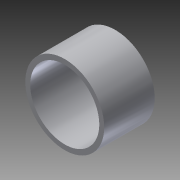
# Autodesk Inventor part: Spacer (0.4375 ID whatever OD) aluminum
Saved by Autodesk Inventor 2014 (Build 180170000, 170)
## iProperties
Created: 2014-01-20
Part Number: Spacer (0.4375 ID whatever OD) aluminum
Material: Aluminum 6061
Document SubType Name: Modeling
Designer: Andrew Toennies
Mass: 0.653976 g
Surface Area: 6.67429 cm^2
Volume: 0.241319 cm^3
Density: 2.71 g/cm^3
Appearance: Aluminum - Flat
Author: Andrew Toennies
Autodesk Inventor part; units mm, degrees
ref_plane "YZ Plane" through (0, 0, 0) normal (1, 0, 0) x (0, 1, 0)
ref_plane "XZ Plane" through (0, 0, 0) normal (0, 1, 0) x (-1, 0, 0)
ref_plane "XY Plane" through (0, 0, 0) normal (0, 0, 1) x (1, 0, 0)
sketch "Sketch1" plane through (0, 0, 0) normal (0, 0, 1) x (1, 0, 0)
  circle A0 centre (0, 0) radius 5.5563
  circle A1 centre (0, 0) radius 6.35
  dimension "d0" = 11.1125
  dimension "d1" = 12.7
  constraints: 2 centre point, 2 coincident
  measures "d0" diameter of A0
  measures "d1" diameter of A1
extrude "Extrusion1" add sketch "Sketch1" along normal blind 8.128
body "Solid1"
